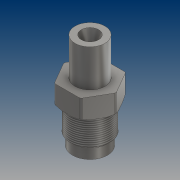
# Autodesk Inventor part: MUSAB1
Saved by Autodesk Inventor 2021 (Build 250183000, 183)
## iProperties
Created: 2017-09-11
Part Number: MUSAB1
Material: Steel, Carbon
Document SubType Name: Modeling
Designer: Amer Mohia
Density: 7.85 g/cm^3
Appearance: Semi-Polished
Author: Amer Mohia
Autodesk Inventor part; units mm, degrees
ref_plane "YZ Plane" through (0, 0, 0) normal (1, 0, 0) x (0, 1, 0)
ref_plane "XZ Plane" through (0, 0, 0) normal (0, 1, 0) x (-1, 0, 0)
sketch "Sketch1" plane through (0, 0, 0) normal (0, 0, 1) x (1, 0, 0)
  line L0 (-5.25, 9.0933) -> (5.25, 9.0933)
  line L1 (5.25, 9.0933) -> (10.5, 0)
  line L2 (10.5, 0) -> (5.25, -9.0933)
  line L3 (5.25, -9.0933) -> (-5.25, -9.0933)
  line L4 (-5.25, -9.0933) -> (-10.5, 0)
  line L5 (-10.5, 0) -> (-5.25, 9.0933)
  point P0 (0, 0)
  point P1 (0, 0)
  dimension "d7" = 21
  constraints: 12 end point, 1 coincident, 13 other
  measures "d7" distance of L1.end L4.end
extrude "Extrusion1" add sketch "Sketch1" along normal blind 8
sketch "Sketch2" plane through (0, 0, 0) normal (0, 1, 0) x (-1, 0, 0)
  line L0 (-5.25, 0) -> (-10.5, 0) projected
  line L1 (-5.25, 0) -> (-5.25, 8) projected
  line L2 (-10.5, 8) -> (-5.25, 8) projected
  line L3 (-10.5, 0) -> (-10.5, 8) projected
  line L4 (10.5, 0) -> (5.25, 0) projected
  line L5 (10.5, 0) -> (10.5, 8) projected
  line L6 (5.25, 8) -> (10.5, 8) projected
  line L7 (5.25, 0) -> (5.25, 8) projected
  line L8 (0, -1.2964) -> (0, 15.0794)
  line L9 (-7.353, 13.0438) -> (-13.5143, 13.0438)
  line L10 (-13.5143, 13.0438) -> (-13.5143, 8.4837)
  line L11 (-13.5143, 8.4837) -> (-7.2541, 13.0438)
  line L12 (-7.2541, 13.0438) -> (-7.353, 13.0438)
  point P0 (0, 0)
  constraints: 10 end point, 1 collinear, 1 horizontal, 1 perpendicular, 1 point on line, 1 vertical
revolve "Revolution1" cut sketch "Sketch2" angle 360 about axis through (0, 0, -1.2964) along (0, 0, 1) contours L12 L11 L10 L9
ref_plane "Work Plane1" through (0, 0, 5.75) normal (0, 0, -1) x (-1, 0, 0)
sketch "Sketch3" plane through (0, 0, 5.75) normal (0, 0, -1) x (-1, 0, 0)
  point P0 (0, 0)
mirror "Mirror1" about plane through (0, 0, 5.75) normal (0, 0, -1) of "Revolution1"
sketch "Sketch4" plane through (0, 0, 8) normal (0, 0, 1) x (1, 0, 0)
  circle A0 centre (0, 0) radius 6
  dimension "d8" = 12
  constraints: 1 centre point, 1 coincident
  measures "d8" diameter of A0
extrude "Extrusion2" add sketch "Sketch4" along normal blind 15
sketch "Sketch5" plane through (0, 0, 23) normal (0, 0, 1) x (1, 0, 0)
  circle A0 centre (0, 0) radius 3.5
  dimension "d11" = 7
  constraints: 1 centre point, 1 coincident
  measures "d11" diameter of A0
extrude "Extrusion3" cut sketch "Sketch5" against normal blind 4
sketch "Sketch6" plane through (0, 0, 19) normal (0, 0, 1) x (1, 0, 0)
  circle A0 centre (0, 0) radius 1.75
  dimension "d14" = 3.5
  constraints: 1 centre point, 1 coincident
  measures "d14" diameter of A0
extrude "Extrusion4" cut sketch "Sketch6" against normal blind 2.5
chamfer "Chamfer1" distance 4 distance2 1.75 1 edges at (-3.5, 0, 19) measured on face at (-3.5, 0, 19.5)
sketch "Sketch7" plane through (0, 0, 0) normal (0, 0, -1) x (-1, 0, 0)
  circle A0 centre (0, 0) radius 8
  dimension "d20" = 16
  constraints: 1 centre point, 1 coincident
  measures "d20" diameter of A0
extrude "Extrusion5" add sketch "Sketch7" along normal blind 10.5
sketch "Sketch8" plane through (0, 0, -10.5) normal (0, 0, -1) x (-1, 0, 0)
  circle A0 centre (0, 0) radius 7
  dimension "d23" = 14
  constraints: 1 centre point, 1 coincident
  measures "d23" diameter of A0
extrude "Extrusion6" add sketch "Sketch8" along normal blind 5
fillet "Fillet1" radius 1 1 edges at (7, 0, -10.5)
thread "Thread1"
sketch "Sketch9" plane through (0, 0, -15.5) normal (0, 0, -1) x (-1, 0, 0)
  circle A0 centre (0, 0) radius 4
  dimension "d29" = 8
  constraints: 1 centre point, 1 coincident
  measures "d29" diameter of A0
extrude "Extrusion7" cut sketch "Sketch9" against normal blind 15
sketch "Sketch10" plane through (0, 0, 0) normal (0, 1, 0) x (-1, 0, 0)
  line L0 (-2.2749, 11.5) -> (-6.7376, 11.5) projected
  line L1 (4, -15.5) -> (4, -0.5) projected
  line L2 (8.8538, 11.5) -> (4, -4.2646)
  line L3 (8.069, 11.5) -> (3.6924, -2.7148)
  line L4 (4, -4.2646) -> (3.6924, -2.7148)
  line L5 (8.8538, 11.5) -> (8.069, 11.5)
  point P0 (0, 0)
  dimension "d32" = 0.75
  constraints: 8 end point, 3 point on line, 1 horizontal, 1 parallel
  measures "d32" distance between parallel lines of L3 L2
revolve "Revolution2" cut sketch "Sketch10" angle 360 about axis through (-8.069, 0, 11.5) along (0.2942595, 0, -0.9557255)
sketch "Sketch11" plane through (0, 0, 0) normal (0, 1, 0) x (-1, 0, 0)
  line L0 (-1.75, 16.5) -> (1.75, 16.5) projected
  line L1 (0, 16.5) -> (-5.6653, 0)
  line L2 (8, 0) -> (-8, 0) projected
  line L3 (-5.6653, 0) -> (-5.6653, -25.3564)
  line L4 (-5.6653, -25.3564) -> (-5.6653, -27.3598)
  point P0 (0, 0)
  constraints: 6 end point, 2 vertical, 1 midpoint, 1 point on line
sketch "Sketch12" plane through (0, 0, 16.5) normal (0, 0, 1) x (1, 0, 0)
  circle A0 centre (0, 0) radius 0.75
  dimension "d34" = 1.5
  constraints: 1 centre point, 1 coincident
  measures "d34" diameter of A0
sweep "Sweep1" cut profiles "Sketch12" path "Sketch11" path curves L1 L3 L4
fillet "Fillet2" radius 1 6 edges at (5.25, -9.0933, 4.4103) (10.5, 0, 4.4103) (5.25, 9.0933, 4.4103) (-5.25, -9.0933, 4.4103) (-5.25, 9.0933, 4.4103) (-10.5, 0, 4.4103)
body "Solid1"
